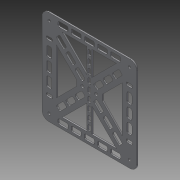
# Autodesk Inventor part: piastraY
Saved by Autodesk Inventor 2014 SP1 (Build 180222100, 222)
## iProperties
Created: 2015-04-08
Part Number: piastraY
Material: Generic
Document SubType Name: Modeling
Designer: Giorgio Nuzzo
Density: 1 g/cm^3
Appearance: Default
Author: Giorgio Nuzzo
Autodesk Inventor part; units mm, degrees
(part 1 of 4)
ref_plane "YZ Plane" through (0, 0, 0) normal (1, 0, 0) x (0, 1, 0)
ref_plane "XZ Plane" through (0, 0, 0) normal (0, 1, 0) x (-1, 0, 0)
ref_plane "XY Plane" through (0, 0, 0) normal (0, 0, 1) x (1, 0, 0)
sketch "Sketch1" plane through (0, 0, 0) normal (0, 1, 0) x (-1, 0, 0)
  line L0 (-63.1017, -60.9985) -> (-63.0908, -60.7839)
  line L1 (-63.0908, -60.7839) -> (-63.0589, -60.5751)
  line L2 (-63.0589, -60.5751) -> (-63.0073, -60.3739)
  line L3 (-63.0073, -60.3739) -> (-62.9366, -60.181)
  line L4 (-62.9366, -60.181) -> (-62.8483, -59.9974)
  line L5 (-62.8483, -59.9974) -> (-62.743, -59.8244)
  line L6 (-62.743, -59.8244) -> (-62.6221, -59.6629)
  line L7 (-62.6221, -59.6629) -> (-62.4865, -59.5137)
  line L8 (-62.4865, -59.5137) -> (-62.3375, -59.3779)
  line L9 (-62.3375, -59.3779) -> (-62.1758, -59.257)
  line L10 (-62.1758, -59.257) -> (-62.0027, -59.1519)
  line L11 (-62.0027, -59.1519) -> (-61.8191, -59.0634)
  line L12 (-61.8191, -59.0634) -> (-61.6261, -58.9928)
  line L13 (-61.6261, -58.9928) -> (-61.4249, -58.9411)
  line L14 (-61.4249, -58.9411) -> (-61.2163, -58.9094)
  line L15 (-61.2163, -58.9094) -> (-61.0017, -58.8984)
  line L16 (-61.0017, -58.8984) -> (-60.7869, -58.9094)
  line L17 (-60.7869, -58.9094) -> (-60.5785, -58.9411)
  line L18 (-60.5785, -58.9411) -> (-60.3773, -58.9928)
  line L19 (-60.3773, -58.9928) -> (-60.1844, -59.0634)
  line L20 (-60.1844, -59.0634) -> (-60.0007, -59.1519)
  line L21 (-60.0007, -59.1519) -> (-59.8276, -59.257)
  line L22 (-59.8276, -59.257) -> (-59.6659, -59.3779)
  line L23 (-59.6659, -59.3779) -> (-59.5167, -59.5137)
  line L24 (-59.5167, -59.5137) -> (-59.3813, -59.6629)
  line L25 (-59.3813, -59.6629) -> (-59.2604, -59.8244)
  line L26 (-59.2604, -59.8244) -> (-59.1551, -59.9974)
  line L27 (-59.1551, -59.9974) -> (-59.0668, -60.181)
  line L28 (-59.0668, -60.181) -> (-58.9961, -60.3739)
  line L29 (-58.9961, -60.3739) -> (-58.9443, -60.5751)
  line L30 (-58.9443, -60.5751) -> (-58.9126, -60.7839)
  line L31 (-58.9126, -60.7839) -> (-58.9017, -60.9985)
  line L32 (-58.9017, -60.9985) -> (-58.9126, -61.2131)
  line L33 (-58.9126, -61.2131) -> (-58.9443, -61.4216)
  line L34 (-58.9443, -61.4216) -> (-58.9961, -61.6231)
  line L35 (-58.9961, -61.6231) -> (-59.0668, -61.816)
  line L36 (-59.0668, -61.816) -> (-59.1551, -61.9993)
  line L37 (-59.1551, -61.9993) -> (-59.2604, -62.1726)
  line L38 (-59.2604, -62.1726) -> (-59.3813, -62.3342)
  line L39 (-59.3813, -62.3342) -> (-59.5167, -62.4834)
  line L40 (-59.5167, -62.4834) -> (-59.6659, -62.6191)
  line L41 (-59.6659, -62.6191) -> (-59.8276, -62.74)
  line L42 (-59.8276, -62.74) -> (-60.0007, -62.8451)
  line L43 (-60.0007, -62.8451) -> (-60.1844, -62.9336)
  line L44 (-60.1844, -62.9336) -> (-60.3773, -63.0039)
  line L45 (-60.3773, -63.0039) -> (-60.5785, -63.0559)
  line L46 (-60.5785, -63.0559) -> (-60.7869, -63.0876)
  line L47 (-60.7869, -63.0876) -> (-61.0017, -63.0986)
  line L48 (-61.0017, -63.0986) -> (-61.2163, -63.0876)
  line L49 (-61.2163, -63.0876) -> (-61.4249, -63.0559)
  line L50 (-61.4249, -63.0559) -> (-61.6261, -63.0039)
  line L51 (-61.6261, -63.0039) -> (-61.8191, -62.9336)
  line L52 (-61.8191, -62.9336) -> (-62.0027, -62.8451)
  line L53 (-62.0027, -62.8451) -> (-62.1758, -62.74)
  line L54 (-62.1758, -62.74) -> (-62.3375, -62.6191)
  line L55 (-62.3375, -62.6191) -> (-62.4865, -62.4834)
  line L56 (-62.4865, -62.4834) -> (-62.6221, -62.3342)
  line L57 (-62.6221, -62.3342) -> (-62.743, -62.1726)
  line L58 (-62.743, -62.1726) -> (-62.8483, -61.9993)
  line L59 (-62.8483, -61.9993) -> (-62.9366, -61.816)
  line L60 (-62.9366, -61.816) -> (-63.0073, -61.6231)
  line L61 (-63.0073, -61.6231) -> (-63.0589, -61.4216)
  line L62 (-63.0589, -61.4216) -> (-63.0908, -61.2131)
  line L63 (-63.0908, -61.2131) -> (-63.1017, -60.9985)
  line L64 (60.6532, 71.991) -> (60.6643, 71.9911)
  line L65 (-61.3617, 71.9911) -> (-61.3543, 71.9911)
  line L66 (-61.3543, 71.9911) -> (-60.7068, 71.9911)
  line L67 (-60.7068, 71.9911) -> (-60.6291, 71.9911)
  line L68 (-60.6291, 71.9911) -> (-51.3537, 71.9911)
  line L69 (-51.3537, 71.9911) -> (-51.3449, 71.9911)
  line L70 (-51.3449, 71.9911) -> (51.3515, 71.9911)
  line L71 (51.3515, 71.9911) -> (51.4421, 71.9911)
  line L72 (51.4421, 71.9911) -> (60.6643, 71.9911)
  line L73 (60.6643, 71.9911) -> (60.728, 71.9911)
  line L74 (60.728, 71.9911) -> (60.7518, 71.9911)
  line L75 (60.7518, 71.9911) -> (61.3543, 71.9911)
  line L76 (61.3543, 71.9911) -> (61.5166, 71.9853)
  line L77 (61.5166, 71.9853) -> (62.1515, 71.9376)
  line L78 (62.1515, 71.9376) -> (62.7826, 71.8533)
  line L79 (62.7826, 71.8533) -> (63.3921, 71.7362)
  line L80 (63.3921, 71.7362) -> (63.9936, 71.5846)
  line L81 (63.9936, 71.5846) -> (64.5858, 71.3993)
  line L82 (64.5858, 71.3993) -> (65.1663, 71.1805)
  line L83 (65.1663, 71.1805) -> (65.6476, 70.9698)
  line L84 (65.6476, 70.9698) -> (66.1182, 70.7361)
  line L85 (66.1182, 70.7361) -> (66.5767, 70.4803)
  line L86 (66.5767, 70.4803) -> (67.0229, 70.2028)
  line L87 (67.0229, 70.2028) -> (67.4552, 69.9044)
  line L88 (67.4552, 69.9044) -> (67.8731, 69.5858)
  line L89 (67.8731, 69.5858) -> (68.2752, 69.2476)
  line L90 (68.2752, 69.2476) -> (68.6603, 68.8905)
  line L91 (68.6603, 68.8905) -> (68.867, 68.6845)
  line L92 (68.867, 68.6845) -> (69.2153, 68.3114)
  line L93 (69.2153, 68.3114) -> (69.5464, 67.9228)
  line L94 (69.5464, 67.9228) -> (69.8585, 67.5189)
  line L95 (69.8585, 67.5189) -> (70.152, 67.1013)
  line L96 (70.152, 67.1013) -> (70.4762, 66.5861)
  line L97 (70.4762, 66.5861) -> (70.7711, 66.0537)
  line L98 (70.7711, 66.0537) -> (71.0361, 65.5059)
  line L99 (71.0361, 65.5059) -> (71.2703, 64.9442)
  line L100 (71.2703, 64.9442) -> (71.475, 64.362)
  line L101 (71.475, 64.362) -> (71.6476, 63.7692)
  line L102 (71.6476, 63.7692) -> (71.7861, 63.1584)
  line L103 (71.7861, 63.1584) -> (71.8915, 62.5409)
  line L104 (71.8915, 62.5409) -> (71.8915, 59.4536)
  line L105 (71.8915, 59.4536) -> (71.8915, 51.721)
  line L106 (71.8915, 51.721) -> (71.8915, 44.999)
  line L107 (71.8915, 44.999) -> (71.8915, 29.9989)
  line L108 (71.8915, 29.9989) -> (71.8915, -29.9985)
  line L109 (71.8915, -29.9985) -> (71.8915, -44.9985)
  line L110 (71.8915, -44.9985) -> (71.8915, -51.7181)
  line L111 (71.8915, -51.7181) -> (71.8915, -59.4565)
  line L112 (71.8915, -59.4565) -> (71.8915, -62.5412)
  line L113 (71.8915, -62.5412) -> (71.8853, -62.5877)
  line L114 (71.8853, -62.5877) -> (71.7898, -63.1465)
  line L115 (71.7898, -63.1465) -> (71.6651, -63.6995)
  line L116 (71.6651, -63.6995) -> (71.5122, -64.2452)
  line L117 (71.5122, -64.2452) -> (71.3316, -64.7823)
  line L118 (71.3316, -64.7823) -> (71.1132, -65.3324)
  line L119 (71.1132, -65.3324) -> (70.8652, -65.8699)
  line L120 (70.8652, -65.8699) -> (70.5882, -66.3932)
  line L121 (70.5882, -66.3932) -> (70.2837, -66.9007)
  line L122 (70.2837, -66.9007) -> (69.9526, -67.3916)
  line L123 (69.9526, -67.3916) -> (69.5953, -67.8636)
  line L124 (69.5953, -67.8636) -> (69.2136, -68.3159)
  line L125 (69.2136, -68.3159) -> (68.8081, -68.7472)
  line L126 (68.8081, -68.7472) -> (68.6896, -68.8633)
  line L127 (68.6896, -68.8633) -> (68.4205, -69.119)
  line L128 (68.4205, -69.119) -> (68.1425, -69.3653)
  line L129 (68.1425, -69.3653) -> (67.7401, -69.6929)
  line L130 (67.7401, -69.6929) -> (67.3229, -70.0016)
  line L131 (67.3229, -70.0016) -> (66.8913, -70.2903)
  line L132 (66.8913, -70.2903) -> (66.4472, -70.5587)
  line L133 (66.4472, -70.5587) -> (65.9322, -70.8343)
  line L134 (65.9322, -70.8343) -> (65.4037, -71.083)
  line L135 (65.4037, -71.083) -> (64.8066, -71.3231)
  line L136 (64.8066, -71.3231) -> (64.1969, -71.5281)
  line L137 (64.1969, -71.5281) -> (63.5761, -71.6966)
  line L138 (63.5761, -71.6966) -> (62.9463, -71.8282)
  line L139 (62.9463, -71.8282) -> (62.362, -71.916)
  line L140 (62.362, -71.916) -> (61.7736, -71.9732)
  line L141 (61.7736, -71.9732) -> (61.6082, -71.9835)
  line L142 (61.6082, -71.9835) -> (61.6051, -71.9835)
  line L143 (61.6051, -71.9835) -> (60.3928, -71.9835)
  line L144 (60.3928, -71.9835) -> (51.348, -71.9835)
  line L145 (51.348, -71.9835) -> (-51.3468, -71.9835)
  line L146 (-51.3468, -71.9835) -> (-60.4217, -71.9835)
  line L147 (-60.4217, -71.9835) -> (-61.5679, -71.9835)
  line L148 (-61.5679, -71.9835) -> (-61.5727, -71.9835)
  line L149 (-61.5727, -71.9835) -> (-61.7421, -71.9736)
  line L150 (-61.7421, -71.9736) -> (-62.3165, -71.9205)
  line L151 (-62.3165, -71.9205) -> (-62.8874, -71.8371)
  line L152 (-62.8874, -71.8371) -> (-63.4531, -71.7238)
  line L153 (-63.4531, -71.7238) -> (-64.0122, -71.5812)
  line L154 (-64.0122, -71.5812) -> (-64.6235, -71.3879)
  line L155 (-64.6235, -71.3879) -> (-65.2225, -71.1591)
  line L156 (-65.2225, -71.1591) -> (-65.8069, -70.8952)
  line L157 (-65.8069, -70.8952) -> (-66.3748, -70.5979)
  line L158 (-66.3748, -70.5979) -> (-66.9247, -70.2682)
  line L159 (-66.9247, -70.2682) -> (-67.4545, -69.9072)
  line L160 (-67.4545, -69.9072) -> (-67.9623, -69.5158)
  line L161 (-67.9623, -69.5158) -> (-68.4464, -69.0955)
  line L162 (-68.4464, -69.0955) -> (-68.8462, -68.7083)
  line L163 (-68.8462, -68.7083) -> (-69.3896, -68.1144)
  line L164 (-69.3896, -68.1144) -> (-69.7224, -67.7027)
  line L165 (-69.7224, -67.7027) -> (-70.0356, -67.2755)
  line L166 (-70.0356, -67.2755) -> (-70.3698, -66.7656)
  line L167 (-70.3698, -66.7656) -> (-70.6752, -66.2382)
  line L168 (-70.6752, -66.2382) -> (-70.9511, -65.6945)
  line L169 (-70.9511, -65.6945) -> (-71.1964, -65.1361)
  line L170 (-71.1964, -65.1361) -> (-71.4117, -64.5576)
  line L171 (-71.4117, -64.5576) -> (-71.5955, -63.9678)
  line L172 (-71.5955, -63.9678) -> (-71.6908, -63.6034)
  line L173 (-71.6908, -63.6034) -> (-71.7714, -63.2358)
  line L174 (-71.7714, -63.2358) -> (-71.8987, -62.4937)
  line L175 (-71.8987, -62.4937) -> (-71.8987, -59.5033)
  line L176 (-71.8987, -59.5033) -> (-71.8987, -51.7298)
  line L177 (-71.8987, -51.7298) -> (-71.8987, -44.9902)
  line L178 (-71.8987, -44.9902) -> (-71.8987, 45.0005)
  line L179 (-71.8987, 45.0005) -> (-71.8987, 51.7279)
  line L180 (-71.8987, 51.7279) -> (-71.8987, 59.502)
  line L181 (-71.8987, 59.502) -> (-71.8987, 62.4925)
  line L182 (-71.8987, 62.4925) -> (-71.8188, 62.9901)
  line L183 (-71.8188, 62.9901) -> (-71.7178, 63.4838)
  line L184 (-71.7178, 63.4838) -> (-71.5601, 64.0848)
  line L185 (-71.5601, 64.0848) -> (-71.3695, 64.676)
  line L186 (-71.3695, 64.676) -> (-71.1489, 65.2465)
  line L187 (-71.1489, 65.2465) -> (-70.8967, 65.8036)
  line L188 (-70.8967, 65.8036) -> (-70.614, 66.3458)
  line L189 (-70.614, 66.3458) -> (-70.3016, 66.8717)
  line L190 (-70.3016, 66.8717) -> (-70.0818, 67.2049)
  line L191 (-70.0818, 67.2049) -> (-69.8508, 67.5304)
  line L192 (-69.8508, 67.5304) -> (-69.5573, 67.9087)
  line L193 (-69.5573, 67.9087) -> (-69.2484, 68.2747)
  line L194 (-69.2484, 68.2747) -> (-68.6987, 68.8533)
  line L195 (-68.6987, 68.8533) -> (-68.3341, 69.1953)
  line L196 (-68.3341, 69.1953) -> (-67.9543, 69.5201)
  line L197 (-67.9543, 69.5201) -> (-67.5601, 69.8274)
  line L198 (-67.5601, 69.8274) -> (-67.1526, 70.1167)
  line L199 (-67.1526, 70.1167) -> (-66.7323, 70.3873)
  line L200 (-66.7323, 70.3873) -> (-66.3001, 70.6384)
  line L201 (-66.3001, 70.6384) -> (-65.857, 70.8696)
  line L202 (-65.857, 70.8696) -> (-65.4038, 71.0802)
  line L203 (-65.4038, 71.0802) -> (-64.8285, 71.3124)
  line L204 (-64.8285, 71.3124) -> (-64.241, 71.5119)
  line L205 (-64.241, 71.5119) -> (-63.6431, 71.6776)
  line L206 (-63.6431, 71.6776) -> (-63.0367, 71.8091)
  line L207 (-63.0367, 71.8091) -> (-62.4087, 71.9078)
  line L208 (-62.4087, 71.9078) -> (-61.776, 71.9706)
  line L209 (-61.776, 71.9706) -> (-61.3881, 71.9901)
  line L210 (-61.3881, 71.9901) -> (-61.3617, 71.9911)
  line L211 (7.9974, -0.0009) -> (8.0104, 0.2548)
  line L212 (8.0104, 0.2548) -> (8.0483, 0.503)
  line L213 (8.0483, 0.503) -> (8.11, 0.7426)
  line L214 (8.11, 0.7426) -> (8.1941, 0.9722)
  line L215 (8.1941, 0.9722) -> (8.2991, 1.1908)
  line L216 (8.2991, 1.1908) -> (8.4246, 1.3968)
  line L217 (8.4246, 1.3968) -> (8.5682, 1.5894)
  line L218 (8.5682, 1.5894) -> (8.7298, 1.7668)
  line L219 (8.7298, 1.7668) -> (8.9072, 1.9282)
  line L220 (8.9072, 1.9282) -> (9.0998, 2.0722)
  line L221 (9.0998, 2.0722) -> (9.3058, 2.1975)
  line L222 (9.3058, 2.1975) -> (9.5246, 2.3027)
  line L223 (9.5246, 2.3027) -> (9.754, 2.3868)
  line L224 (9.754, 2.3868) -> (9.9938, 2.4483)
  line L225 (9.9938, 2.4483) -> (10.2418, 2.4862)
  line L226 (10.2418, 2.4862) -> (10.4975, 2.4991)
  line L227 (10.4975, 2.4991) -> (10.7531, 2.4862)
  line L228 (10.7531, 2.4862) -> (11.0015, 2.4483)
  line L229 (11.0015, 2.4483) -> (11.2409, 2.3868)
  line L230 (11.2409, 2.3868) -> (11.4707, 2.3027)
  line L231 (11.4707, 2.3027) -> (11.6891, 2.1975)
  line L232 (11.6891, 2.1975) -> (11.8951, 2.0722)
  line L233 (11.8951, 2.0722) -> (12.0877, 1.9282)
  line L234 (12.0877, 1.9282) -> (12.2651, 1.7668)
  line L235 (12.2651, 1.7668) -> (12.4267, 1.5894)
  line L236 (12.4267, 1.5894) -> (12.5707, 1.3968)
  line L237 (12.5707, 1.3968) -> (12.6958, 1.1908)
  line L238 (12.6958, 1.1908) -> (12.8012, 0.9722)
  line L239 (12.8012, 0.9722) -> (12.8853, 0.7426)
  line L240 (12.8853, 0.7426) -> (12.9466, 0.503)
  line L241 (12.9466, 0.503) -> (12.9845, 0.2548)
  line L242 (12.9845, 0.2548) -> (12.9976, -0.0009)
  line L243 (12.9976, -0.0009) -> (12.9845, -0.2565)
  line L244 (12.9845, -0.2565) -> (12.9466, -0.5047)
  line L245 (12.9466, -0.5047) -> (12.8853, -0.7443)
  line L246 (12.8853, -0.7443) -> (12.8012, -0.9739)
  line L247 (12.8012, -0.9739) -> (12.6958, -1.1925)
  line L248 (12.6958, -1.1925) -> (12.5707, -1.3987)
  line L249 (12.5707, -1.3987) -> (12.4267, -1.5911)
  line L250 (12.4267, -1.5911) -> (12.2651, -1.7687)
  line L251 (12.2651, -1.7687) -> (12.0877, -1.9299)
  line L252 (12.0877, -1.9299) -> (11.8951, -2.0739)
  line L253 (11.8951, -2.0739) -> (11.6891, -2.1992)
  line L254 (11.6891, -2.1992) -> (11.4707, -2.3044)
  line L255 (11.4707, -2.3044) -> (11.2409, -2.3885)
  line L256 (11.2409, -2.3885) -> (11.0015, -2.4502)
  line L257 (11.0015, -2.4502) -> (10.7531, -2.488)
  line L258 (10.7531, -2.488) -> (10.4975, -2.5008)
  line L259 (10.4975, -2.5008) -> (10.2418, -2.488)
  line L260 (10.2418, -2.488) -> (9.9938, -2.4502)
  line L261 (9.9938, -2.4502) -> (9.754, -2.3885)
  line L262 (9.754, -2.3885) -> (9.5246, -2.3044)
  line L263 (9.5246, -2.3044) -> (9.3058, -2.1992)
  line L264 (9.3058, -2.1992) -> (9.0998, -2.0739)
  line L265 (9.0998, -2.0739) -> (8.9072, -1.9299)
  line L266 (8.9072, -1.9299) -> (8.7298, -1.7687)
  line L267 (8.7298, -1.7687) -> (8.5682, -1.5911)
  line L268 (8.5682, -1.5911) -> (8.4246, -1.3987)
  line L269 (8.4246, -1.3987) -> (8.2991, -1.1925)
  line L270 (8.2991, -1.1925) -> (8.1941, -0.9739)
  line L271 (8.1941, -0.9739) -> (8.11, -0.7443)
  line L272 (8.11, -0.7443) -> (8.0483, -0.5047)
  line L273 (8.0483, -0.5047) -> (8.0104, -0.2565)
  line L274 (8.0104, -0.2565) -> (7.9974, -0.0009)
  line L275 (-13.0012, -0.0009) -> (-12.9883, 0.2548)
  line L276 (-12.9883, 0.2548) -> (-12.9504, 0.503)
  line L277 (-12.9504, 0.503) -> (-12.8887, 0.7426)
  line L278 (-12.8887, 0.7426) -> (-12.8046, 0.9722)
  line L279 (-12.8046, 0.9722) -> (-12.6994, 1.1908)
  line L280 (-12.6994, 1.1908) -> (-12.5742, 1.3968)
  line L281 (-12.5742, 1.3968) -> (-12.4303, 1.5894)
  line L282 (-12.4303, 1.5894) -> (-12.2689, 1.7668)
  line L283 (-12.2689, 1.7668) -> (-12.0913, 1.9282)
  line L284 (-12.0913, 1.9282) -> (-11.8989, 2.0722)
  line L285 (-11.8989, 2.0722) -> (-11.6927, 2.1975)
  line L286 (-11.6927, 2.1975) -> (-11.4743, 2.3027)
  line L287 (-11.4743, 2.3027) -> (-11.2445, 2.3868)
  line L288 (-11.2445, 2.3868) -> (-11.0051, 2.4483)
  line L289 (-11.0051, 2.4483) -> (-10.7567, 2.4862)
  line L290 (-10.7567, 2.4862) -> (-10.5013, 2.4991)
  line L291 (-10.5013, 2.4991) -> (-10.2456, 2.4862)
  line L292 (-10.2456, 2.4862) -> (-9.9974, 2.4483)
  line L293 (-9.9974, 2.4483) -> (-9.7578, 2.3868)
  line L294 (-9.7578, 2.3868) -> (-9.528, 2.3027)
  line L295 (-9.528, 2.3027) -> (-9.3096, 2.1975)
  line L296 (-9.3096, 2.1975) -> (-9.1034, 2.0722)
  line L297 (-9.1034, 2.0722) -> (-8.911, 1.9282)
  line L298 (-8.911, 1.9282) -> (-8.7334, 1.7668)
  line L299 (-8.7334, 1.7668) -> (-8.572, 1.5894)
  line L300 (-8.572, 1.5894) -> (-8.4282, 1.3968)
  line L301 (-8.4282, 1.3968) -> (-8.3029, 1.1908)
  line L302 (-8.3029, 1.1908) -> (-8.1977, 0.9722)
  line L303 (-8.1977, 0.9722) -> (-8.1136, 0.7426)
  line L304 (-8.1136, 0.7426) -> (-8.052, 0.503)
  line L305 (-8.052, 0.503) -> (-8.0141, 0.2548)
  line L306 (-8.0141, 0.2548) -> (-8.0011, -0.0009)
  line L307 (-8.0011, -0.0009) -> (-8.0141, -0.2565)
  line L308 (-8.0141, -0.2565) -> (-8.052, -0.5047)
  line L309 (-8.052, -0.5047) -> (-8.1136, -0.7443)
  line L310 (-8.1136, -0.7443) -> (-8.1977, -0.9739)
  line L311 (-8.1977, -0.9739) -> (-8.3029, -1.1925)
  line L312 (-8.3029, -1.1925) -> (-8.4282, -1.3987)
  line L313 (-8.4282, -1.3987) -> (-8.572, -1.5911)
  line L314 (-8.572, -1.5911) -> (-8.7334, -1.7687)
  line L315 (-8.7334, -1.7687) -> (-8.911, -1.9299)
  line L316 (-8.911, -1.9299) -> (-9.1034, -2.0739)
  line L317 (-9.1034, -2.0739) -> (-9.3096, -2.1992)
  line L318 (-9.3096, -2.1992) -> (-9.528, -2.3044)
  line L319 (-9.528, -2.3044) -> (-9.7578, -2.3885)
  line L320 (-9.7578, -2.3885) -> (-9.9974, -2.4502)
  line L321 (-9.9974, -2.4502) -> (-10.2456, -2.488)
  line L322 (-10.2456, -2.488) -> (-10.5013, -2.5008)
  line L323 (-10.5013, -2.5008) -> (-10.7567, -2.488)
  line L324 (-10.7567, -2.488) -> (-11.0051, -2.4502)
  line L325 (-11.0051, -2.4502) -> (-11.2445, -2.3885)
  line L326 (-11.2445, -2.3885) -> (-11.4743, -2.3044)
  line L327 (-11.4743, -2.3044) -> (-11.6927, -2.1992)
  line L328 (-11.6927, -2.1992) -> (-11.8989, -2.0739)
  line L329 (-11.8989, -2.0739) -> (-12.0913, -1.9299)
  line L330 (-12.0913, -1.9299) -> (-12.2689, -1.7687)
  line L331 (-12.2689, -1.7687) -> (-12.4303, -1.5911)
  line L332 (-12.4303, -1.5911) -> (-12.5742, -1.3987)
  line L333 (-12.5742, -1.3987) -> (-12.6994, -1.1925)
  line L334 (-12.6994, -1.1925) -> (-12.8046, -0.9739)
  line L335 (-12.8046, -0.9739) -> (-12.8887, -0.7443)
  line L336 (-12.8887, -0.7443) -> (-12.9504, -0.5047)
  line L337 (-12.9504, -0.5047) -> (-12.9883, -0.2565)
  line L338 (-12.9883, -0.2565) -> (-13.0012, -0.0009)
  spline S0 degree 3 poles (-65.0013, -37.5233) (-65.0013, -38.9041) (-63.8821, -40.0234) (-62.5014, -40.0234) knots 0 0 0 0 1 1 1 1
  line L339 (-65.0013, -37.5233) -> (-65.0013, -38.9041) construction
  line L340 (-65.0013, -38.9041) -> (-63.8821, -40.0234) construction
  line L341 (-63.8821, -40.0234) -> (-62.5014, -40.0234) construction
  line L342 (-62.5014, -40.0234) -> (-59.5014, -40.0234)
  spline S1 degree 3 poles (-59.5014, -40.0234) (-58.1206, -40.0234) (-57.0014, -38.9041) (-57.0014, -37.5233) knots 2 2 2 2 3 3 3 3
  line L343 (-59.5014, -40.0234) -> (-58.1206, -40.0234) construction
  line L344 (-58.1206, -40.0234) -> (-57.0014, -38.9041) construction
  line L345 (-57.0014, -38.9041) -> (-57.0014, -37.5233) construction
  line L346 (-57.0014, -37.5233) -> (-57.0014, -37.4733)
  spline S2 degree 3 poles (-57.0014, -37.4733) (-57.0014, -36.0925) (-58.1206, -34.9732) (-59.5014, -34.9732) knots 4 4 4 4 5 5 5 5
  line L347 (-57.0014, -37.4733) -> (-57.0014, -36.0925) construction
  line L348 (-57.0014, -36.0925) -> (-58.1206, -34.9732) construction
  line L349 (-58.1206, -34.9732) -> (-59.5014, -34.9732) construction
  line L350 (-59.5014, -34.9732) -> (-62.5014, -34.9732)
  spline S3 degree 3 poles (-62.5014, -34.9732) (-63.8821, -34.9732) (-65.0013, -36.0925) (-65.0013, -37.4733) knots 6 6 6 6 7 7 7 7
  line L351 (-62.5014, -34.9732) -> (-63.8821, -34.9732) construction
  line L352 (-63.8821, -34.9732) -> (-65.0013, -36.0925) construction
  line L353 (-65.0013, -36.0925) -> (-65.0013, -37.4733) construction
  line L354 (-65.0013, -37.4733) -> (-65.0013, -37.5233)
  spline S4 degree 3 poles (-65.0015, 37.4752) (-65.0015, 36.0946) (-63.8821, 34.9753) (-62.5015, 34.9753) knots 0 0 0 0 1 1 1 1
  line L355 (-65.0015, 37.4752) -> (-65.0015, 36.0946) construction
  line L356 (-65.0015, 36.0946) -> (-63.8821, 34.9753) construction
  line L357 (-63.8821, 34.9753) -> (-62.5015, 34.9753) construction
  line L358 (-62.5015, 34.9753) -> (-59.5014, 34.9753)
  spline S5 degree 3 poles (-59.5014, 34.9753) (-58.1207, 34.9753) (-57.0014, 36.0946) (-57.0014, 37.4752) knots 2 2 2 2 3 3 3 3
  line L359 (-59.5014, 34.9753) -> (-58.1207, 34.9753) construction
  line L360 (-58.1207, 34.9753) -> (-57.0014, 36.0946) construction
  line L361 (-57.0014, 36.0946) -> (-57.0014, 37.4752) construction
  line L362 (-57.0014, 37.4752) -> (-57.0014, 37.5254)
  spline S6 degree 3 poles (-57.0014, 37.5254) (-57.0014, 38.906) (-58.1207, 40.0253) (-59.5014, 40.0253) knots 4 4 4 4 5 5 5 5
  line L363 (-57.0014, 37.5254) -> (-57.0014, 38.906) construction
  line L364 (-57.0014, 38.906) -> (-58.1207, 40.0253) construction
  line L365 (-58.1207, 40.0253) -> (-59.5014, 40.0253) construction
  line L366 (-59.5014, 40.0253) -> (-62.5015, 40.0253)
  spline S7 degree 3 poles (-62.5015, 40.0253) (-63.8821, 40.0253) (-65.0015, 38.906) (-65.0015, 37.5254) knots 6 6 6 6 7 7 7 7
  line L367 (-62.5015, 40.0253) -> (-63.8821, 40.0253) construction
  line L368 (-63.8821, 40.0253) -> (-65.0015, 38.906) construction
  line L369 (-65.0015, 38.906) -> (-65.0015, 37.5254) construction
  line L370 (-65.0015, 37.5254) -> (-65.0015, 37.4752)
  spline S8 degree 3 poles (55.9993, 37.4757) (55.9993, 36.0951) (57.1186, 34.9758) (58.4994, 34.9758) knots 0 0 0 0 1 1 1 1
  line L371 (55.9993, 37.4757) -> (55.9993, 36.0951) construction
  line L372 (55.9993, 36.0951) -> (57.1186, 34.9758) construction
  line L373 (57.1186, 34.9758) -> (58.4994, 34.9758) construction
  line L374 (58.4994, 34.9758) -> (63.4992, 34.9758)
  spline S9 degree 3 poles (63.4992, 34.9758) (64.88, 34.9758) (65.9993, 36.0951) (65.9993, 37.4757) knots 2 2 2 2 3 3 3 3
  line L375 (63.4992, 34.9758) -> (64.88, 34.9758) construction
  line L376 (64.88, 34.9758) -> (65.9993, 36.0951) construction
  line L377 (65.9993, 36.0951) -> (65.9993, 37.4757) construction
  line L378 (65.9993, 37.4757) -> (65.9993, 37.5259)
  spline S10 degree 3 poles (65.9993, 37.5259) (65.9993, 38.9065) (64.88, 40.0258) (63.4992, 40.0258) knots 4 4 4 4 5 5 5 5
  line L379 (65.9993, 37.5259) -> (65.9993, 38.9065) construction
  line L380 (65.9993, 38.9065) -> (64.88, 40.0258) construction
  line L381 (64.88, 40.0258) -> (63.4992, 40.0258) construction
  line L382 (63.4992, 40.0258) -> (58.4994, 40.0258)
  spline S11 degree 3 poles (58.4994, 40.0258) (57.1186, 40.0258) (55.9993, 38.9065) (55.9993, 37.5259) knots 6 6 6 6 7 7 7 7
  line L383 (58.4994, 40.0258) -> (57.1186, 40.0258) construction
  line L384 (57.1186, 40.0258) -> (55.9993, 38.9065) construction
  line L385 (55.9993, 38.9065) -> (55.9993, 37.5259) construction
  line L386 (55.9993, 37.5259) -> (55.9993, 37.4757)
  spline S12 degree 3 poles (55.9993, -37.5212) (55.9993, -38.902) (57.1186, -40.0213) (58.4994, -40.0213) knots 0 0 0 0 1 1 1 1
  line L387 (55.9993, -37.5212) -> (55.9993, -38.902) construction
  line L388 (55.9993, -38.902) -> (57.1186, -40.0213) construction
  line L389 (57.1186, -40.0213) -> (58.4994, -40.0213) construction
  line L390 (58.4994, -40.0213) -> (63.4992, -40.0213)
  spline S13 degree 3 poles (63.4992, -40.0213) (64.88, -40.0213) (65.9993, -38.902) (65.9993, -37.5212) knots 2 2 2 2 3 3 3 3
  line L391 (63.4992, -40.0213) -> (64.88, -40.0213) construction
  line L392 (64.88, -40.0213) -> (65.9993, -38.902) construction
  line L393 (65.9993, -38.902) -> (65.9993, -37.5212) construction
  line L394 (65.9993, -37.5212) -> (65.9993, -37.4713)
  spline S14 degree 3 poles (65.9993, -37.4713) (65.9993, -36.0905) (64.88, -34.9712) (63.4992, -34.9712) knots 4 4 4 4 5 5 5 5
  line L395 (65.9993, -37.4713) -> (65.9993, -36.0905) construction
  line L396 (65.9993, -36.0905) -> (64.88, -34.9712) construction
  line L397 (64.88, -34.9712) -> (63.4992, -34.9712) construction
  line L398 (63.4992, -34.9712) -> (58.4994, -34.9712)
  spline S15 degree 3 poles (58.4994, -34.9712) (57.1186, -34.9712) (55.9993, -36.0905) (55.9993, -37.4713) knots 6 6 6 6 7 7 7 7
  line L399 (58.4994, -34.9712) -> (57.1186, -34.9712) construction
  line L400 (57.1186, -34.9712) -> (55.9993, -36.0905) construction
  line L401 (55.9993, -36.0905) -> (55.9993, -37.4713) construction
  line L402 (55.9993, -37.4713) -> (55.9993, -37.5212)
  line L403 (19.3996, -4.4032) -> (19.3996, -4.0004)
  line L404 (19.3996, -4.0004) -> (19.3996, 3.9996)
  line L405 (19.3996, 3.9996) -> (19.3996, 4.4418)
  line L406 (19.3996, 4.4418) -> (50.0055, 35.0476)
  line L407 (50.0055, 35.0476) -> (50.0055, 3.9996)
  line L408 (50.0055, 3.9996) -> (50.0055, -4.0004)
  line L409 (50.0055, -4.0004) -> (50.0055, -35.0091)
  line L410 (50.0055, -35.0091) -> (19.3996, -4.4032)
  line L411 (-19.4514, 4.453) -> (-50.007, 35.0084)
  line L412 (-50.007, 35.0084) -> (-50.007, -4.0004)
  line L413 (-50.007, -4.0004) -> (-50.007, -35.0077)
  line L414 (-50.007, -35.0077) -> (-49.8933, -34.894)
  line L415 (-49.8933, -34.894) -> (-32.575, -17.5757)
  line L416 (-32.575, -17.5757) -> (-19.4514, -4.4521)
  line L417 (-19.4514, -4.4521) -> (-19.4514, -4.0004)
  line L418 (-19.4514, -4.0004) -> (-19.4514, 3.9996)
  line L419 (-19.4514, 3.9996) -> (-19.4514, 4.453)
  line L420 (-41.1585, 56.1578) -> (-3.9986, 56.1578)
  line L421 (-3.9986, 56.1578) -> (-3.9986, 18.9801)
  line L422 (-3.9986, 18.9801) -> (-32.575, 47.5563)
  line L423 (-32.575, 47.5563) -> (-41.1674, 56.1487)
  line L424 (-41.1674, 56.1487) -> (-41.1585, 56.1578)
  line L425 (41.1357, 56.1578) -> (4.0012, 56.1578)
  line L426 (4.0012, 56.1578) -> (4.0012, 19.0231)
  line L427 (4.0012, 19.0231) -> (41.1357, 56.1578)
  line L428 (-41.1514, -56.0179) -> (-32.575, -47.4417)
  line L429 (-32.575, -47.4417) -> (-3.9986, -18.8653)
  line L430 (-3.9986, -18.8653) -> (-3.9986, -56.0179)
  line L431 (-3.9986, -56.0179) -> (-41.1514, -56.0179)
  line L432 (4.0012, -56.0179) -> (4.0012, -18.9084)
  line L433 (4.0012, -18.9084) -> (41.1109, -56.0179)
  line L434 (41.1109, -56.0179) -> (4.0012, -56.0179)
  spline S16 degree 3 poles (45.3977, -67.8667) (46.6754, -67.8667) (47.7114, -66.8307) (47.7114, -65.5529) knots 0 0 0 0 1 1 1 1
  line L435 (45.3977, -67.8667) -> (46.6754, -67.8667) construction
  line L436 (46.6754, -67.8667) -> (47.7114, -66.8307) construction
  line L437 (47.7114, -66.8307) -> (47.7114, -65.5529) construction
  line L438 (47.7114, -65.5529) -> (47.7114, -62.4678)
  spline S17 degree 3 poles (47.7114, -62.4678) (47.7114, -61.1901) (46.6754, -60.1541) (45.3977, -60.1541) knots 2 2 2 2 3 3 3 3
  line L439 (47.7114, -62.4678) -> (47.7114, -61.1901) construction
  line L440 (47.7114, -61.1901) -> (46.6754, -60.1541) construction
  line L441 (46.6754, -60.1541) -> (45.3977, -60.1541) construction
  line L442 (45.3977, -60.1541) -> (34.6, -60.1541)
  spline S18 degree 3 poles (34.6, -60.1541) (33.3223, -60.1541) (32.2863, -61.1901) (32.2863, -62.4678) knots 4 4 4 4 5 5 5 5
  line L443 (34.6, -60.1541) -> (33.3223, -60.1541) construction
  line L444 (33.3223, -60.1541) -> (32.2863, -61.1901) construction
  line L445 (32.2863, -61.1901) -> (32.2863, -62.4678) construction
  line L446 (32.2863, -62.4678) -> (32.2863, -65.5529)
  spline S19 degree 3 poles (32.2863, -65.5529) (32.2863, -66.8307) (33.3223, -67.8667) (34.6, -67.8667) knots 6 6 6 6 7 7 7 7
  line L447 (32.2863, -65.5529) -> (32.2863, -66.8307) construction
  line L448 (32.2863, -66.8307) -> (33.3223, -67.8667) construction
  line L449 (33.3223, -67.8667) -> (34.6, -67.8667) construction
  line L450 (34.6, -67.8667) -> (45.3977, -67.8667)
  spline S20 degree 3 poles (25.3975, -67.8667) (26.6753, -67.8667) (27.7112, -66.8307) (27.7112, -65.5529) knots 0 0 0 0 1 1 1 1
  line L451 (25.3975, -67.8667) -> (26.6753, -67.8667) construction
  line L452 (26.6753, -67.8667) -> (27.7112, -66.8307) construction
  line L453 (27.7112, -66.8307) -> (27.7112, -65.5529) construction
  line L454 (27.7112, -65.5529) -> (27.7112, -62.4678)
  spline S21 degree 3 poles (27.7112, -62.4678) (27.7112, -61.1901) (26.6753, -60.1541) (25.3975, -60.1541) knots 2 2 2 2 3 3 3 3
  line L455 (27.7112, -62.4678) -> (27.7112, -61.1901) construction
  line L456 (27.7112, -61.1901) -> (26.6753, -60.1541) construction
  line L457 (26.6753, -60.1541) -> (25.3975, -60.1541) construction
  line L458 (25.3975, -60.1541) -> (14.5999, -60.1541)
  spline S22 degree 3 poles (14.5999, -60.1541) (13.3221, -60.1541) (12.2862, -61.1901) (12.2862, -62.4678) knots 4 4 4 4 5 5 5 5
  line L459 (14.5999, -60.1541) -> (13.3221, -60.1541) construction
  line L460 (13.3221, -60.1541) -> (12.2862, -61.1901) construction
  line L461 (12.2862, -61.1901) -> (12.2862, -62.4678) construction
  line L462 (12.2862, -62.4678) -> (12.2862, -65.5529)
  spline S23 degree 3 poles (12.2862, -65.5529) (12.2862, -66.8307) (13.3221, -67.8667) (14.5999, -67.8667) knots 6 6 6 6 7 7 7 7
  line L463 (12.2862, -65.5529) -> (12.2862, -66.8307) construction
  line L464 (12.2862, -66.8307) -> (13.3221, -67.8667) construction
  line L465 (13.3221, -67.8667) -> (14.5999, -67.8667) construction
  line L466 (14.5999, -67.8667) -> (25.3975, -67.8667)
  spline S24 degree 3 poles (5.3975, -67.8667) (6.6755, -67.8667) (7.7114, -66.8307) (7.7114, -65.5529) knots 0 0 0 0 1 1 1 1
  line L467 (5.3975, -67.8667) -> (6.6755, -67.8667) construction
  line L468 (6.6755, -67.8667) -> (7.7114, -66.8307) construction
  line L469 (7.7114, -66.8307) -> (7.7114, -65.5529) construction
  line L470 (7.7114, -65.5529) -> (7.7114, -62.4678)
  spline S25 degree 3 poles (7.7114, -62.4678) (7.7114, -61.1901) (6.6755, -60.1541) (5.3975, -60.1541) knots 2 2 2 2 3 3 3 3
  line L471 (7.7114, -62.4678) -> (7.7114, -61.1901) construction
  line L472 (7.7114, -61.1901) -> (6.6755, -60.1541) construction
  line L473 (6.6755, -60.1541) -> (5.3975, -60.1541) construction
  line L474 (5.3975, -60.1541) -> (-5.4001, -60.1541)
  spline S26 degree 3 poles (-5.4001, -60.1541) (-6.6779, -60.1541) (-7.7138, -61.1901) (-7.7138, -62.4678) knots 4 4 4 4 5 5 5 5
  line L475 (-5.4001, -60.1541) -> (-6.6779, -60.1541) construction
  line L476 (-6.6779, -60.1541) -> (-7.7138, -61.1901) construction
  line L477 (-7.7138, -61.1901) -> (-7.7138, -62.4678) construction
  line L478 (-7.7138, -62.4678) -> (-7.7138, -65.5529)
  spline S27 degree 3 poles (-7.7138, -65.5529) (-7.7138, -66.8307) (-6.6779, -67.8667) (-5.4001, -67.8667) knots 6 6 6 6 7 7 7 7
  line L479 (-7.7138, -65.5529) -> (-7.7138, -66.8307) construction
  line L480 (-7.7138, -66.8307) -> (-6.6779, -67.8667) construction
  line L481 (-6.6779, -67.8667) -> (-5.4001, -67.8667) construction
  line L482 (-5.4001, -67.8667) -> (5.3975, -67.8667)
  spline S28 degree 3 poles (-14.6025, -67.8667) (-13.3247, -67.8667) (-12.2887, -66.8307) (-12.2887, -65.5529) knots 0 0 0 0 1 1 1 1
  line L483 (-14.6025, -67.8667) -> (-13.3247, -67.8667) construction
  line L484 (-13.3247, -67.8667) -> (-12.2887, -66.8307) construction
  line L485 (-12.2887, -66.8307) -> (-12.2887, -65.5529) construction
  line L486 (-12.2887, -65.5529) -> (-12.2887, -62.4678)
  spline S29 degree 3 poles (-12.2887, -62.4678) (-12.2887, -61.1901) (-13.3247, -60.1541) (-14.6025, -60.1541) knots 2 2 2 2 3 3 3 3
  line L487 (-12.2887, -62.4678) -> (-12.2887, -61.1901) construction
  line L488 (-12.2887, -61.1901) -> (-13.3247, -60.1541) construction
  line L489 (-13.3247, -60.1541) -> (-14.6025, -60.1541) construction
  line L490 (-14.6025, -60.1541) -> (-25.4001, -60.1541)
  spline S30 degree 3 poles (-25.4001, -60.1541) (-26.6779, -60.1541) (-27.7138, -61.1901) (-27.7138, -62.4678) knots 4 4 4 4 5 5 5 5
  line L491 (-25.4001, -60.1541) -> (-26.6779, -60.1541) construction
  line L492 (-26.6779, -60.1541) -> (-27.7138, -61.1901) construction
  line L493 (-27.7138, -61.1901) -> (-27.7138, -62.4678) construction
  line L494 (-27.7138, -62.4678) -> (-27.7138, -65.5529)
  spline S31 degree 3 poles (-27.7138, -65.5529) (-27.7138, -66.8307) (-26.6779, -67.8667) (-25.4001, -67.8667) knots 6 6 6 6 7 7 7 7
  line L495 (-27.7138, -65.5529) -> (-27.7138, -66.8307) construction
  line L496 (-27.7138, -66.8307) -> (-26.6779, -67.8667) construction
  line L497 (-26.6779, -67.8667) -> (-25.4001, -67.8667) construction
  line L498 (-25.4001, -67.8667) -> (-14.6025, -67.8667)
  spline S32 degree 3 poles (-34.6025, -67.8667) (-33.3247, -67.8667) (-32.2887, -66.8307) (-32.2887, -65.5529) knots 0 0 0 0 1 1 1 1
  line L499 (-34.6025, -67.8667) -> (-33.3247, -67.8667) construction
  line L500 (-33.3247, -67.8667) -> (-32.2887, -66.8307) construction
  line L501 (-32.2887, -66.8307) -> (-32.2887, -65.5529) construction
  line L502 (-32.2887, -65.5529) -> (-32.2887, -62.4678)
  spline S33 degree 3 poles (-32.2887, -62.4678) (-32.2887, -61.1901) (-33.3247, -60.1541) (-34.6025, -60.1541) knots 2 2 2 2 3 3 3 3
  line L503 (-32.2887, -62.4678) -> (-32.2887, -61.1901) construction
  line L504 (-32.2887, -61.1901) -> (-33.3247, -60.1541) construction
  line L505 (-33.3247, -60.1541) -> (-34.6025, -60.1541) construction
  line L506 (-34.6025, -60.1541) -> (-45.4001, -60.1541)
  spline S34 degree 3 poles (-45.4001, -60.1541) (-46.6779, -60.1541) (-47.7138, -61.1901) (-47.7138, -62.4678) knots 4 4 4 4 5 5 5 5
  line L507 (-45.4001, -60.1541) -> (-46.6779, -60.1541) construction
  line L508 (-46.6779, -60.1541) -> (-47.7138, -61.1901) construction
  line L509 (-47.7138, -61.1901) -> (-47.7138, -62.4678) construction
  line L510 (-47.7138, -62.4678) -> (-47.7138, -65.5529)
  spline S35 degree 3 poles (-47.7138, -65.5529) (-47.7138, -66.8307) (-46.6779, -67.8667) (-45.4001, -67.8667) knots 6 6 6 6 7 7 7 7
  line L511 (-47.7138, -65.5529) -> (-47.7138, -66.8307) construction
  line L512 (-47.7138, -66.8307) -> (-46.6779, -67.8667) construction
  line L513 (-46.6779, -67.8667) -> (-45.4001, -67.8667) construction
  line L514 (-45.4001, -67.8667) -> (-34.6025, -67.8667)
  spline S36 degree 3 poles (45.3977, 60.2137) (46.6754, 60.2137) (47.7114, 61.2495) (47.7114, 62.5274) knots 0 0 0 0 1 1 1 1
  line L515 (45.3977, 60.2137) -> (46.6754, 60.2137) construction
  line L516 (46.6754, 60.2137) -> (47.7114, 61.2495) construction
  line L517 (47.7114, 61.2495) -> (47.7114, 62.5274) construction
  line L518 (47.7114, 62.5274) -> (47.7114, 65.6124)
  spline S37 degree 3 poles (47.7114, 65.6124) (47.7114, 66.8903) (46.6754, 67.9263) (45.3977, 67.9263) knots 2 2 2 2 3 3 3 3
  line L519 (47.7114, 65.6124) -> (47.7114, 66.8903) construction
  line L520 (47.7114, 66.8903) -> (46.6754, 67.9263) construction
  line L521 (46.6754, 67.9263) -> (45.3977, 67.9263) construction
  line L522 (45.3977, 67.9263) -> (34.6, 67.9263)
  spline S38 degree 3 poles (34.6, 67.9263) (33.3223, 67.9263) (32.2863, 66.8903) (32.2863, 65.6124) knots 4 4 4 4 5 5 5 5
  line L523 (34.6, 67.9263) -> (33.3223, 67.9263) construction
  line L524 (33.3223, 67.9263) -> (32.2863, 66.8903) construction
  line L525 (32.2863, 66.8903) -> (32.2863, 65.6124) construction
  line L526 (32.2863, 65.6124) -> (32.2863, 62.5274)
  spline S39 degree 3 poles (32.2863, 62.5274) (32.2863, 61.2495) (33.3223, 60.2137) (34.6, 60.2137) knots 6 6 6 6 7 7 7 7
  line L527 (32.2863, 62.5274) -> (32.2863, 61.2495) construction
  line L528 (32.2863, 61.2495) -> (33.3223, 60.2137) construction
  line L529 (33.3223, 60.2137) -> (34.6, 60.2137) construction
  line L530 (34.6, 60.2137) -> (45.3977, 60.2137)
  spline S40 degree 3 poles (25.3975, 60.2137) (26.6753, 60.2137) (27.7112, 61.2495) (27.7112, 62.5274) knots 0 0 0 0 1 1 1 1
  line L531 (25.3975, 60.2137) -> (26.6753, 60.2137) construction
  line L532 (26.6753, 60.2137) -> (27.7112, 61.2495) construction
  line L533 (27.7112, 61.2495) -> (27.7112, 62.5274) construction
  line L534 (27.7112, 62.5274) -> (27.7112, 65.6124)
  spline S41 degree 3 poles (27.7112, 65.6124) (27.7112, 66.8903) (26.6753, 67.9263) (25.3975, 67.9263) knots 2 2 2 2 3 3 3 3
  line L535 (27.7112, 65.6124) -> (27.7112, 66.8903) construction
  line L536 (27.7112, 66.8903) -> (26.6753, 67.9263) construction
  line L537 (26.6753, 67.9263) -> (25.3975, 67.9263) construction
  line L538 (25.3975, 67.9263) -> (14.5999, 67.9263)
  spline S42 degree 3 poles (14.5999, 67.9263) (13.3221, 67.9263) (12.2862, 66.8903) (12.2862, 65.6124) knots 4 4 4 4 5 5 5 5
  line L539 (14.5999, 67.9263) -> (13.3221, 67.9263) construction
  line L540 (13.3221, 67.9263) -> (12.2862, 66.8903) construction
  line L541 (12.2862, 66.8903) -> (12.2862, 65.6124) construction
  line L542 (12.2862, 65.6124) -> (12.2862, 62.5274)
  spline S43 degree 3 poles (12.2862, 62.5274) (12.2862, 61.2495) (13.3221, 60.2137) (14.5999, 60.2137) knots 6 6 6 6 7 7 7 7
  line L543 (12.2862, 62.5274) -> (12.2862, 61.2495) construction
  line L544 (12.2862, 61.2495) -> (13.3221, 60.2137) construction
  line L545 (13.3221, 60.2137) -> (14.5999, 60.2137) construction
  line L546 (14.5999, 60.2137) -> (25.3975, 60.2137)
  spline S44 degree 3 poles (5.3975, 60.2137) (6.6755, 60.2137) (7.7114, 61.2495) (7.7114, 62.5274) knots 0 0 0 0 1 1 1 1
  line L547 (5.3975, 60.2137) -> (6.6755, 60.2137) construction
  line L548 (6.6755, 60.2137) -> (7.7114, 61.2495) construction
  line L549 (7.7114, 61.2495) -> (7.7114, 62.5274) construction
  line L550 (7.7114, 62.5274) -> (7.7114, 65.6124)
  spline S45 degree 3 poles (7.7114, 65.6124) (7.7114, 66.8903) (6.6755, 67.9263) (5.3975, 67.9263) knots 2 2 2 2 3 3 3 3
  line L551 (7.7114, 65.6124) -> (7.7114, 66.8903) construction
  line L552 (7.7114, 66.8903) -> (6.6755, 67.9263) construction
  line L553 (6.6755, 67.9263) -> (5.3975, 67.9263) construction
  line L554 (5.3975, 67.9263) -> (-5.4001, 67.9263)
  spline S46 degree 3 poles (-5.4001, 67.9263) (-6.6779, 67.9263) (-7.7138, 66.8903) (-7.7138, 65.6124) knots 4 4 4 4 5 5 5 5
  line L555 (-5.4001, 67.9263) -> (-6.6779, 67.9263) construction
  line L556 (-6.6779, 67.9263) -> (-7.7138, 66.8903) construction
  line L557 (-7.7138, 66.8903) -> (-7.7138, 65.6124) construction
  line L558 (-7.7138, 65.6124) -> (-7.7138, 62.5274)
  spline S47 degree 3 poles (-7.7138, 62.5274) (-7.7138, 61.2495) (-6.6779, 60.2137) (-5.4001, 60.2137) knots 6 6 6 6 7 7 7 7
  line L559 (-7.7138, 62.5274) -> (-7.7138, 61.2495) construction
  line L560 (-7.7138, 61.2495) -> (-6.6779, 60.2137) construction
  line L561 (-6.6779, 60.2137) -> (-5.4001, 60.2137) construction
  line L562 (-5.4001, 60.2137) -> (5.3975, 60.2137)
  spline S48 degree 3 poles (-14.6025, 60.2137) (-13.3247, 60.2137) (-12.2887, 61.2495) (-12.2887, 62.5274) knots 0 0 0 0 1 1 1 1
  line L563 (-14.6025, 60.2137) -> (-13.3247, 60.2137) construction
  line L564 (-13.3247, 60.2137) -> (-12.2887, 61.2495) construction
  line L565 (-12.2887, 61.2495) -> (-12.2887, 62.5274) construction
  line L566 (-12.2887, 62.5274) -> (-12.2887, 65.6124)
  spline S49 degree 3 poles (-12.2887, 65.6124) (-12.2887, 66.8903) (-13.3247, 67.9263) (-14.6025, 67.9263) knots 2 2 2 2 3 3 3 3
  line L567 (-12.2887, 65.6124) -> (-12.2887, 66.8903) construction
  line L568 (-12.2887, 66.8903) -> (-13.3247, 67.9263) construction
  line L569 (-13.3247, 67.9263) -> (-14.6025, 67.9263) construction
  line L570 (-14.6025, 67.9263) -> (-25.4001, 67.9263)
  spline S50 degree 3 poles (-25.4001, 67.9263) (-26.6779, 67.9263) (-27.7138, 66.8903) (-27.7138, 65.6124) knots 4 4 4 4 5 5 5 5
  line L571 (-25.4001, 67.9263) -> (-26.6779, 67.9263) construction
  line L572 (-26.6779, 67.9263) -> (-27.7138, 66.8903) construction
  line L573 (-27.7138, 66.8903) -> (-27.7138, 65.6124) construction
  line L574 (-27.7138, 65.6124) -> (-27.7138, 62.5274)
  spline S51 degree 3 poles (-27.7138, 62.5274) (-27.7138, 61.2495) (-26.6779, 60.2137) (-25.4001, 60.2137) knots 6 6 6 6 7 7 7 7
  line L575 (-27.7138, 62.5274) -> (-27.7138, 61.2495) construction
  line L576 (-27.7138, 61.2495) -> (-26.6779, 60.2137) construction
  line L577 (-26.6779, 60.2137) -> (-25.4001, 60.2137) construction
  line L578 (-25.4001, 60.2137) -> (-14.6025, 60.2137)
  spline S52 degree 3 poles (-34.6025, 60.2137) (-33.3247, 60.2137) (-32.2887, 61.2495) (-32.2887, 62.5274) knots 0 0 0 0 1 1 1 1
  line L579 (-34.6025, 60.2137) -> (-33.3247, 60.2137) construction
  line L580 (-33.3247, 60.2137) -> (-32.2887, 61.2495) construction
  line L581 (-32.2887, 61.2495) -> (-32.2887, 62.5274) construction
  line L582 (-32.2887, 62.5274) -> (-32.2887, 65.6124)
  spline S53 degree 3 poles (-32.2887, 65.6124) (-32.2887, 66.8903) (-33.3247, 67.9263) (-34.6025, 67.9263) knots 2 2 2 2 3 3 3 3
  line L583 (-32.2887, 65.6124) -> (-32.2887, 66.8903) construction
  line L584 (-32.2887, 66.8903) -> (-33.3247, 67.9263) construction
  line L585 (-33.3247, 67.9263) -> (-34.6025, 67.9263) construction
  line L586 (-34.6025, 67.9263) -> (-45.4001, 67.9263)
  spline S54 degree 3 poles (-45.4001, 67.9263) (-46.6779, 67.9263) (-47.7138, 66.8903) (-47.7138, 65.6124) knots 4 4 4 4 5 5 5 5
  line L587 (-45.4001, 67.9263) -> (-46.6779, 67.9263) construction
  line L588 (-46.6779, 67.9263) -> (-47.7138, 66.8903) construction
  line L589 (-47.7138, 66.8903) -> (-47.7138, 65.6124) construction
  line L590 (-47.7138, 65.6124) -> (-47.7138, 62.5274)
  spline S55 degree 3 poles (-47.7138, 62.5274) (-47.7138, 61.2495) (-46.6779, 60.2137) (-45.4001, 60.2137) knots 6 6 6 6 7 7 7 7
  line L591 (-47.7138, 62.5274) -> (-47.7138, 61.2495) construction
  line L592 (-47.7138, 61.2495) -> (-46.6779, 60.2137) construction
  line L593 (-46.6779, 60.2137) -> (-45.4001, 60.2137) construction
  line L594 (-45.4001, 60.2137) -> (-34.6025, 60.2137)
  spline S56 degree 3 poles (-2.0682, 46.7406) (-2.0682, 46.0552) (-1.5127, 45.4997) (-0.8273, 45.4997) knots 0 0 0 0 1 1 1 1
  line L595 (-2.0682, 46.7406) -> (-2.0682, 46.0552) construction
  line L596 (-2.0682, 46.0552) -> (-1.5127, 45.4997) construction
  line L597 (-1.5127, 45.4997) -> (-0.8273, 45.4997) construction
  line L598 (-0.8273, 45.4997) -> (0.8273, 45.4997)
  spline S57 degree 3 poles (0.8273, 45.4997) (1.5125, 45.4997) (2.0682, 46.0552) (2.0682, 46.7406) knots 2 2 2 2 3 3 3 3
  line L599 (0.8273, 45.4997) -> (1.5125, 45.4997) construction
  line L600 (1.5125, 45.4997) -> (2.0682, 46.0552) construction
  line L601 (2.0682, 46.0552) -> (2.0682, 46.7406) construction
  line L602 (2.0682, 46.7406) -> (2.0682, 52.5315)
  spline S58 degree 3 poles (2.0682, 52.5315) (2.0682, 53.2167) (1.5125, 53.7724) (0.8273, 53.7724) knots 4 4 4 4 5 5 5 5
  line L603 (2.0682, 52.5315) -> (2.0682, 53.2167) construction
  line L604 (2.0682, 53.2167) -> (1.5125, 53.7724) construction
  line L605 (1.5125, 53.7724) -> (0.8273, 53.7724) construction
  line L606 (0.8273, 53.7724) -> (-0.8273, 53.7724)
  spline S59 degree 3 poles (-0.8273, 53.7724) (-1.5127, 53.7724) (-2.0682, 53.2167) (-2.0682, 52.5315) knots 6 6 6 6 7 7 7 7
  line L607 (-0.8273, 53.7724) -> (-1.5127, 53.7724) construction
  line L608 (-1.5127, 53.7724) -> (-2.0682, 53.2167) construction
  line L609 (-2.0682, 53.2167) -> (-2.0682, 52.5315) construction
  line L610 (-2.0682, 52.5315) -> (-2.0682, 46.7406)
  spline S60 degree 3 poles (-2.0682, 34.3316) (-2.0682, 33.6462) (-1.5127, 33.0907) (-0.8273, 33.0907) knots 0 0 0 0 1 1 1 1
  line L611 (-2.0682, 34.3316) -> (-2.0682, 33.6462) construction
  line L612 (-2.0682, 33.6462) -> (-1.5127, 33.0907) construction
  line L613 (-1.5127, 33.0907) -> (-0.8273, 33.0907) construction
  line L614 (-0.8273, 33.0907) -> (0.8273, 33.0907)
  spline S61 degree 3 poles (0.8273, 33.0907) (1.5125, 33.0907) (2.0682, 33.6462) (2.0682, 34.3316) knots 2 2 2 2 3 3 3 3
  line L615 (0.8273, 33.0907) -> (1.5125, 33.0907) construction
  line L616 (1.5125, 33.0907) -> (2.0682, 33.6462) construction
  line L617 (2.0682, 33.6462) -> (2.0682, 34.3316) construction
  line L618 (2.0682, 34.3316) -> (2.0682, 40.1224)
  spline S62 degree 3 poles (2.0682, 40.1224) (2.0682, 40.8078) (1.5125, 41.3634) (0.8273, 41.3634) knots 4 4 4 4 5 5 5 5
  line L619 (2.0682, 40.1224) -> (2.0682, 40.8078) construction
  line L620 (2.0682, 40.8078) -> (1.5125, 41.3634) construction
  line L621 (1.5125, 41.3634) -> (0.8273, 41.3634) construction
  line L622 (0.8273, 41.3634) -> (-0.8273, 41.3634)
  spline S63 degree 3 poles (-0.8273, 41.3634) (-1.5127, 41.3634) (-2.0682, 40.8078) (-2.0682, 40.1224) knots 6 6 6 6 7 7 7 7
  line L623 (-0.8273, 41.3634) -> (-1.5127, 41.3634) construction
  line L624 (-1.5127, 41.3634) -> (-2.0682, 40.8078) construction
  line L625 (-2.0682, 40.8078) -> (-2.0682, 40.1224) construction
  line L626 (-2.0682, 40.1224) -> (-2.0682, 34.3316)
  spline S64 degree 3 poles (-2.0682, 21.9225) (-2.0682, 21.2373) (-1.5127, 20.6816) (-0.8273, 20.6816) knots 0 0 0 0 1 1 1 1
  line L627 (-2.0682, 21.9225) -> (-2.0682, 21.2373) construction
  line L628 (-2.0682, 21.2373) -> (-1.5127, 20.6816) construction
  line L629 (-1.5127, 20.6816) -> (-0.8273, 20.6816) construction
  line L630 (-0.8273, 20.6816) -> (0.8273, 20.6816)
  spline S65 degree 3 poles (0.8273, 20.6816) (1.5125, 20.6816) (2.0682, 21.2373) (2.0682, 21.9225) knots 2 2 2 2 3 3 3 3
  line L631 (0.8273, 20.6816) -> (1.5125, 20.6816) construction
  line L632 (1.5125, 20.6816) -> (2.0682, 21.2373) construction
  line L633 (2.0682, 21.2373) -> (2.0682, 21.9225) construction
  line L634 (2.0682, 21.9225) -> (2.0682, 27.7134)
  spline S66 degree 3 poles (2.0682, 27.7134) (2.0682, 28.3988) (1.5125, 28.9543) (0.8273, 28.9543) knots 4 4 4 4 5 5 5 5
  line L635 (2.0682, 27.7134) -> (2.0682, 28.3988) construction
  line L636 (2.0682, 28.3988) -> (1.5125, 28.9543) construction
  line L637 (1.5125, 28.9543) -> (0.8273, 28.9543) construction
  line L638 (0.8273, 28.9543) -> (-0.8273, 28.9543)
  spline S67 degree 3 poles (-0.8273, 28.9543) (-1.5127, 28.9543) (-2.0682, 28.3988) (-2.0682, 27.7134) knots 6 6 6 6 7 7 7 7
  line L639 (-0.8273, 28.9543) -> (-1.5127, 28.9543) construction
  line L640 (-1.5127, 28.9543) -> (-2.0682, 28.3988) construction
  line L641 (-2.0682, 28.3988) -> (-2.0682, 27.7134) construction
  line L642 (-2.0682, 27.7134) -> (-2.0682, 21.9225)
  spline S68 degree 3 poles (-2.0682, 9.5135) (-2.0682, 8.8282) (-1.5127, 8.2727) (-0.8273, 8.2727) knots 0 0 0 0 1 1 1 1
  line L643 (-2.0682, 9.5135) -> (-2.0682, 8.8282) construction
  line L644 (-2.0682, 8.8282) -> (-1.5127, 8.2727) construction
  line L645 (-1.5127, 8.2727) -> (-0.8273, 8.2727) construction
  line L646 (-0.8273, 8.2727) -> (0.8273, 8.2727)
  spline S69 degree 3 poles (0.8273, 8.2727) (1.5125, 8.2727) (2.0682, 8.8282) (2.0682, 9.5135) knots 2 2 2 2 3 3 3 3
  line L647 (0.8273, 8.2727) -> (1.5125, 8.2727) construction
  line L648 (1.5125, 8.2727) -> (2.0682, 8.8282) construction
  line L649 (2.0682, 8.8282) -> (2.0682, 9.5135) construction
  line L650 (2.0682, 9.5135) -> (2.0682, 15.3045)
  spline S70 degree 3 poles (2.0682, 15.3045) (2.0682, 15.9897) (1.5125, 16.5452) (0.8273, 16.5452) knots 4 4 4 4 5 5 5 5
  line L651 (2.0682, 15.3045) -> (2.0682, 15.9897) construction
  line L652 (2.0682, 15.9897) -> (1.5125, 16.5452) construction
  line L653 (1.5125, 16.5452) -> (0.8273, 16.5452) construction
  line L654 (0.8273, 16.5452) -> (-0.8273, 16.5452)
  spline S71 degree 3 poles (-0.8273, 16.5452) (-1.5127, 16.5452) (-2.0682, 15.9897) (-2.0682, 15.3045) knots 6 6 6 6 7 7 7 7
  line L655 (-0.8273, 16.5452) -> (-1.5127, 16.5452) construction
  line L656 (-1.5127, 16.5452) -> (-2.0682, 15.9897) construction
  line L657 (-2.0682, 15.9897) -> (-2.0682, 15.3045) construction
  line L658 (-2.0682, 15.3045) -> (-2.0682, 9.5135)
  spline S72 degree 3 poles (-2.0682, -2.8954) (-2.0682, -3.5808) (-1.5127, -4.1364) (-0.8273, -4.1364) knots 0 0 0 0 1 1 1 1
  line L659 (-2.0682, -2.8954) -> (-2.0682, -3.5808) construction
  line L660 (-2.0682, -3.5808) -> (-1.5127, -4.1364) construction
  line L661 (-1.5127, -4.1364) -> (-0.8273, -4.1364) construction
  line L662 (-0.8273, -4.1364) -> (0.8273, -4.1364)
  spline S73 degree 3 poles (0.8273, -4.1364) (1.5125, -4.1364) (2.0682, -3.5808) (2.0682, -2.8954) knots 2 2 2 2 3 3 3 3
  line L663 (0.8273, -4.1364) -> (1.5125, -4.1364) construction
  line L664 (1.5125, -4.1364) -> (2.0682, -3.5808) construction
  line L665 (2.0682, -3.5808) -> (2.0682, -2.8954) construction
  line L666 (2.0682, -2.8954) -> (2.0682, 2.8954)
  spline S74 degree 3 poles (2.0682, 2.8954) (2.0682, 3.5807) (1.5125, 4.1364) (0.8273, 4.1364) knots 4 4 4 4 5 5 5 5
  line L667 (2.0682, 2.8954) -> (2.0682, 3.5807) construction
  line L668 (2.0682, 3.5807) -> (1.5125, 4.1364) construction
  line L669 (1.5125, 4.1364) -> (0.8273, 4.1364) construction
  line L670 (0.8273, 4.1364) -> (-0.8273, 4.1364)
  spline S75 degree 3 poles (-0.8273, 4.1364) (-1.5127, 4.1364) (-2.0682, 3.5807) (-2.0682, 2.8954) knots 6 6 6 6 7 7 7 7
  line L671 (-0.8273, 4.1364) -> (-1.5127, 4.1364) construction
  line L672 (-1.5127, 4.1364) -> (-2.0682, 3.5807) construction
  line L673 (-2.0682, 3.5807) -> (-2.0682, 2.8954) construction
  line L674 (-2.0682, 2.8954) -> (-2.0682, -2.8954)
  spline S76 degree 3 poles (-2.0682, -15.3045) (-2.0682, -15.9899) (-1.5127, -16.5454) (-0.8273, -16.5454) knots 0 0 0 0 1 1 1 1
  line L675 (-2.0682, -15.3045) -> (-2.0682, -15.9899) construction
  line L676 (-2.0682, -15.9899) -> (-1.5127, -16.5454) construction
  line L677 (-1.5127, -16.5454) -> (-0.8273, -16.5454) construction
  line L678 (-0.8273, -16.5454) -> (0.8273, -16.5454)